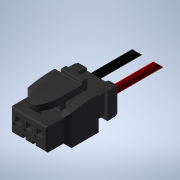
# Autodesk Inventor part: 566654 NEBV-H1G2-KN-0.5-N-LE2
Saved by Autodesk Inventor 2021 (Build 250183000, 183)
## iProperties
Created: 2026-04-16
Part Number: 566654 NEBV-H1G2-KN-0.5-N-LE2
Material: Generic
Catalog Web Link: www.3dfindit.com
Description: NEBV-Connecting cables for valve terminals
Vendor: FESTO
Document SubType Name: Modeling
Designer: psAdmin
Manufacturer: FESTO
Mass: 4 g
Surface Area: 6.95901 cm^2
Volume: 0.50983 cm^3
Density: 1 g/cm^3
Appearance: PSOLRGB-176-176-176
Category: PARTsolutions
Company: FESTO
Title: 566654 NEBV-H1G2-KN-0.5-N-LE2
Author: Cadenas PARTsolutions
Comments: Connecting cables for valve terminals
PSOL_IDENT_0: {$CADENAS_DATA/23d-libs/festo/parts/n/nebv/nebv.prj},197 {VTYP=3D},{NB=566654 NEBV-H1G2-KN-0.5-N-LE2
PSOL_IDENT_1: },{LINA=566654 NEBV-H1G2-KN-0.5-N-LE2},{NN=NEBV},{DATE=23.10.2025 07:10:51},{GEOMDATE=23.10.2025 07:
PSOL_IDENT_2: 10:27},{VERSION=},{LINEID=410},{WBVAR=},{WBNUMERIC=}  {NB=566654 NEBV-H1G2-KN-0.5-N-LE2},{LINA=56665
PSOL_IDENT_3: 4 NEBV-H1G2-KN-0.5-N-LE2},{KT=DUMMY},{TNR=566654},{TYP=NEBV-H1G2-KN-0.5-N-LE2},{INFO=},{KD=0.000},{M
PSOL_IDENT_4: P=-},{L1=0.500},{L2=-},{L3=0.000},{L4=-},{VERS=8},{CNSMASSEXACT=0.0040},{ISASM=0},{PIN=-},{EOLDATE=}
PSOL_IDENT_5: ,{GTIN=4052568057312}
NB: 566654 NEBV-H1G2-KN-0.5-N-LE2
NN: NEBV
NT: Connecting cables for valve terminals
NBSYN: $TNR. $TYP.
LINA: 566654 NEBV-H1G2-KN-0.5-N-LE2
CATALOG: Festo
TNR: 566654
TYP: NEBV-H1G2-KN-0.5-N-LE2
KD: 0
L1: 0.5
L2: -
L3: 0.000
L4: -
CNSMASSEXACT: 0.004
GTIN: 4052568057312
SUPPLIER: FESTO
ARTICLENO: 566654 NEBV-H1G2-KN-0.5-N-LE2
BOMINFO: 566654 NEBV-H1G2-KN-0.5-N-LE2
CREATOR: CADENAS GmbH
Autodesk Inventor part; units mm, degrees
sketch "Sketch_9" plane through (0, 0, 0) normal (1, 0, 0) x (0, 1, 0)
  line L0 (1.4, 13) -> (-2.4, 13)
  line L1 (-2.4, 13) -> (-2.6, 12.8)
  line L2 (-2.6, 12.8) -> (-2.6, 9.85)
  line L3 (-2.6, 9.85) -> (-3.35, 9.1)
  line L4 (-3.35, 9.1) -> (-3.35, 4)
  line L5 (-3.35, 4) -> (-2.07, 4)
  line L6 (-2.07, 4) -> (-2.07, 2)
  line L7 (-2.07, 2) -> (-2.67, 2)
  line L8 (-2.67, 2) -> (-2.6438, 0.5)
  line L9 (-2.6438, 0.5) -> (-2.5098, 0)
  line L10 (-2.5098, 0) -> (2.0698, 0)
  line L11 (2.0698, 0) -> (2.2038, 0.5)
  line L12 (2.2038, 0.5) -> (2.23, 2)
  line L13 (2.23, 2) -> (1.6, 2)
  line L14 (1.6, 2) -> (1.6, 4)
  line L15 (1.6, 4) -> (2.9, 4)
  arc A0 (2.9, 4) -> (2.35, 9.1) centre (-18.6885, 4.2515) ccw
  line L16 (2.35, 9.1) -> (1.6, 9.85)
  line L17 (1.6, 9.85) -> (1.6, 12.8)
  line L18 (1.6, 12.8) -> (1.4, 13)
  constraints: 38 end point, 2 point on circle, 1 centre point
extrude "Extrusion1" add sketch "Sketch_9" along normal mid plane 8.3
sketch "Sketch_23" plane through (0, 0, 0) normal (0, 1, 0) x (-1, 0, 0)
  line L0 (5, 14) -> (-5, 14)
  line L1 (-5, 14) -> (-5, -1)
  line L2 (-5, -1) -> (5, -1)
  line L3 (5, -1) -> (5, 14)
  line L4 (4.13, 9.1) -> (3.38, 9.85)
  line L5 (3.38, 9.85) -> (3.38, 12.8)
  line L6 (3.38, 12.8) -> (3.18, 13)
  line L7 (3.18, 13) -> (-3.18, 13)
  line L8 (-3.18, 13) -> (-3.38, 12.8)
  line L9 (-3.38, 12.8) -> (-3.38, 9.85)
  line L10 (-3.38, 9.85) -> (-4.13, 9.1)
  line L11 (-4.13, 9.1) -> (-4.13, 4)
  line L12 (-4.13, 4) -> (-3.185, 4)
  line L13 (-3.185, 4) -> (-3.185, 2)
  line L14 (-3.185, 2) -> (-3.8, 2)
  line L15 (-3.8, 2) -> (-3.7738, 0.5)
  line L16 (-3.7738, 0.5) -> (-3.6398, 0)
  line L17 (-3.6398, 0) -> (3.6398, 0)
  line L18 (3.6398, 0) -> (3.7738, 0.5)
  line L19 (3.7738, 0.5) -> (3.8, 2)
  line L20 (3.8, 2) -> (3.185, 2)
  line L21 (3.185, 2) -> (3.185, 4)
  line L22 (3.185, 4) -> (4.13, 4)
  line L23 (4.13, 4) -> (4.13, 9.1)
  constraints: 48 end point
extrude "Extrusion2" cut sketch "Sketch_23" along normal mid plane 12
sketch "Sketch_1" plane through (0, 1.6, 0) normal (0, 1, 0) x (1, 0, 0)
  line L0 (-2.8, -4) -> (-2.8, -13)
  line L1 (-2.8, -13) -> (2.8, -13)
  line L2 (2.8, -13) -> (2.8, -4)
  line L3 (2.8, -4) -> (2.04, -4)
  line L4 (2.04, -4) -> (2.04, 0)
  line L5 (2.04, 0) -> (-2.04, 0)
  line L6 (-2.04, 0) -> (-2.04, -4)
  line L7 (-2.04, -4) -> (-2.8, -4)
  constraints: 16 end point
extrude "Extrusion3" cut sketch "Sketch_1" along normal blind 2
sketch "Sketch_2" plane through (0, 0, 0) normal (1, 0, 0) x (0, 1, 0)
  line L0 (3.3881, 12.51) -> (2.87, 12.51)
  line L1 (2.87, 12.51) -> (1.8, 11.6122)
  line L2 (1.8, 11.6122) -> (1.8, 11.3122)
  line L3 (1.8, 11.3122) -> (2.3653, 11.4118)
  arc A0 (2.6, 11.2149) -> (2.3653, 11.4118) centre (2.4, 11.2149) ccw
  line L4 (2.6, 11.2149) -> (2.6, 9.35)
  arc A1 (2.35, 9.1) -> (2.6, 9.35) centre (2.35, 9.35) ccw
  line L5 (2.35, 9.1) -> (1.85, 9.1)
  arc A2 (1.6, 9.35) -> (1.85, 9.1) centre (1.85, 9.35) ccw
  line L6 (1.6, 9.35) -> (0.6, 9.35)
  line L7 (0.6, 9.35) -> (0.6, 7.75)
  line L8 (0.6, 7.75) -> (1.6, 7.75)
  arc A3 (1.95, 8.1) -> (1.6, 7.75) centre (1.95, 7.75) ccw
  line L9 (1.95, 8.1) -> (2.25, 8.1)
  arc A4 (2.6, 7.75) -> (2.25, 8.1) centre (2.25, 7.75) ccw
  line L10 (2.6, 7.75) -> (2.6, 4)
  line L11 (2.6, 4) -> (4.45, 4)
  line L12 (4.45, 4) -> (4.45, 4.8)
  arc A5 (4.45, 4.8) -> (4.25, 5) centre (4.25, 4.8) ccw
  line L13 (4.25, 5) -> (4, 5)
  arc A6 (3.85, 5.15) -> (4, 5) centre (4, 5.15) ccw
  line L14 (3.85, 5.15) -> (3.85, 9.1)
  arc A7 (3.85, 9.1) -> (3.5854, 12.3424) centre (-16.15, 9.1) ccw
  arc A8 (3.5854, 12.3424) -> (3.3881, 12.51) centre (3.3881, 12.31) ccw
  constraints: 30 end point, 18 point on circle, 9 centre point
extrude "Extrusion4" add sketch "Sketch_2" along normal mid plane 4
sketch "Sketch_3" plane through (0, 1.6, 0) normal (0, 1, 0) x (1, 0, 0)
  line L0 (-2.2, -12.8) -> (2.2, -12.8)
  line L1 (2.2, -12.8) -> (2.2, -3.8)
  line L2 (2.2, -3.8) -> (-2.2, -3.8)
  line L3 (-2.2, -3.8) -> (-2.2, -12.8)
  arc A0 (-2, -9.1) -> (-1.1898, -11.8286) centre (3, -9.1) ccw
  arc A1 (-1.1898, -11.8286) -> (1.1898, -11.8286) centre (0, -11.11) ccw
  arc A2 (1.1898, -11.8286) -> (2, -9.1) centre (-3, -9.1) ccw
  line L4 (2, -9.1) -> (2, -4)
  line L5 (2, -4) -> (-2, -4)
  line L6 (-2, -4) -> (-2, -9.1)
  constraints: 14 end point, 6 point on circle, 3 centre point
extrude "Extrusion5" cut sketch "Sketch_3" along normal blind 3
sketch "Sketch_4" plane through (0, 1.6, 0) normal (0, 1, 0) x (1, 0, 0)
  line L0 (-2, -10.5) -> (-2, -13)
  line L1 (-2, -13) -> (-0.765, -13)
  line L2 (-0.765, -13) -> (-0.765, -10.7)
  line L3 (-0.765, -10.7) -> (0.765, -10.7)
  line L4 (0.765, -10.7) -> (0.765, -13)
  line L5 (0.765, -13) -> (2, -13)
  line L6 (2, -13) -> (2, -10.5)
  line L7 (2, -10.5) -> (0.765, -10.5)
  line L8 (0.765, -10.5) -> (0.765, -4)
  line L9 (0.765, -4) -> (2, -4)
  line L10 (2, -4) -> (2, -3)
  line L11 (2, -3) -> (-2, -3)
  line L12 (-2, -3) -> (-2, -4)
  line L13 (-2, -4) -> (-0.765, -4)
  line L14 (-0.765, -4) -> (-0.765, -10.5)
  line L15 (-0.765, -10.5) -> (-2, -10.5)
  constraints: 32 end point
extrude "Extrusion6" cut sketch "Sketch_4" along normal blind 1
sketch "Sketch_5" plane through (0, 0, 4) normal (0, 0, 1) x (1, 0, 0)
  line L0 (-2.3, -3.35) -> (-2.1906, -3.35)
  arc A0 (-1.9953, -3.5068) -> (-2.1906, -3.35) centre (-2.1906, -3.55) ccw
  arc A1 (-1.9953, -3.5068) -> (-1.8621, -3.6537) centre (-1.8, -3.4636) ccw
  arc A2 (-1.8621, -3.6537) -> (1.8621, -3.6537) centre (0, 2.05) ccw
  arc A3 (1.8621, -3.6537) -> (1.9953, -3.5068) centre (1.8, -3.4636) ccw
  arc A4 (2.1906, -3.35) -> (1.9953, -3.5068) centre (2.1906, -3.55) ccw
  line L1 (2.1906, -3.35) -> (2.3, -3.35)
  line L2 (2.3, -3.35) -> (2, 0)
  line L3 (2, 0) -> (-2, 0)
  line L4 (-2, 0) -> (-2.3, -3.35)
  constraints: 10 end point, 10 point on circle, 5 centre point
extrude "Extrusion7" add sketch "Sketch_5" along normal blind 1
sketch "Sketch_6" plane through (0, 0, 9.85) normal (0, 0, 1) x (1, 0, 0)
  line L0 (-1.275, -1.81) -> (-1.275, -3.41)
  line L1 (-1.275, -3.41) -> (1.275, -3.41)
  line L2 (1.275, -3.41) -> (1.275, -1.81)
  line L3 (1.275, -1.81) -> (0.625, -1.81)
  line L4 (0.625, -1.81) -> (0.625, -2.61)
  line L5 (0.625, -2.61) -> (-0.625, -2.61)
  line L6 (-0.625, -2.61) -> (-0.625, -1.81)
  line L7 (-0.625, -1.81) -> (-1.275, -1.81)
  constraints: 16 end point
extrude "Extrusion8" cut sketch "Sketch_6" along normal blind 3.2
sketch "Sketch_19" plane through (0, 0, 13) normal (0, 0, 1) x (1, 0, 0)
  line L0 (-2.4, 0.39) -> (-2.4, -0.41)
  line L1 (-2.4, -0.41) -> (-1.6, -0.41)
  line L2 (-1.6, -0.41) -> (-1.6, 0.39)
  line L3 (-1.6, 0.39) -> (-2.4, 0.39)
  constraints: 8 end point
extrude "Extrusion9" cut sketch "Sketch_19" against normal blind 2.9
sketch "Sketch_20" plane through (0, 0, 13) normal (0, 0, 1) x (1, 0, 0)
  line L0 (-0.4, 0.39) -> (-0.4, -0.41)
  line L1 (-0.4, -0.41) -> (0.4, -0.41)
  line L2 (0.4, -0.41) -> (0.4, 0.39)
  line L3 (0.4, 0.39) -> (-0.4, 0.39)
  constraints: 8 end point
extrude "Extrusion10" cut sketch "Sketch_20" against normal blind 2.9
sketch "Sketch_21" plane through (0, 0, 13) normal (0, 0, 1) x (1, 0, 0)
  line L0 (1.6, 0.39) -> (1.6, -0.41)
  line L1 (1.6, -0.41) -> (2.4, -0.41)
  line L2 (2.4, -0.41) -> (2.4, 0.39)
  line L3 (2.4, 0.39) -> (1.6, 0.39)
  constraints: 8 end point
extrude "Extrusion11" cut sketch "Sketch_21" against normal blind 2.9
sketch "Sketch_7" plane through (0, 0, 13) normal (0, 0, 1) x (1, 0, 0)
  arc A0 (-2.9964, -0.76) -> (-2.0036, -0.76) centre (-2.5, -0.7) ccw
  line L0 (-2.0036, -0.76) -> (-2.9964, -0.76)
  constraints: 2 end point, 2 point on circle, 1 centre point
extrude "Extrusion12" cut sketch "Sketch_7" against normal blind 2.9
sketch "Sketch_8" plane through (0, 0, 13) normal (0, 0, 1) x (1, 0, 0)
  line L0 (0.0036, 0.76) -> (0.9964, 0.76)
  arc A0 (0.9964, 0.76) -> (0.0036, 0.76) centre (0.5, 0.7) ccw
  constraints: 2 end point, 2 point on circle, 1 centre point
extrude "Extrusion13" cut sketch "Sketch_8" against normal blind 2.9
sketch "Sketch_10" plane through (0, 0, 13) normal (0, 0, 1) x (1, 0, 0)
  line L0 (2.0036, 0.76) -> (2.9964, 0.76)
  arc A0 (2.9964, 0.76) -> (2.0036, 0.76) centre (2.5, 0.7) ccw
  constraints: 2 end point, 2 point on circle, 1 centre point
extrude "Extrusion14" cut sketch "Sketch_10" against normal blind 2.9
sketch "Sketch_11" plane through (0, 0, 13) normal (0, 0, 1) x (1, 0, 0)
  line L0 (-1.9964, 0.76) -> (-1.0036, 0.76)
  arc A0 (-1.0036, 0.76) -> (-1.9964, 0.76) centre (-1.5, 0.7) ccw
  constraints: 2 end point, 2 point on circle, 1 centre point
extrude "Extrusion15" cut sketch "Sketch_11" against normal blind 2.9
sketch "Sketch_12" plane through (0, 0, 13) normal (0, 0, 1) x (1, 0, 0)
  arc A0 (-0.9964, -0.76) -> (-0.0036, -0.76) centre (-0.5, -0.7) ccw
  line L0 (-0.0036, -0.76) -> (-0.9964, -0.76)
  constraints: 2 end point, 2 point on circle, 1 centre point
extrude "Extrusion16" cut sketch "Sketch_12" against normal blind 2.9
sketch "Sketch_13" plane through (0, 0, 13) normal (0, 0, 1) x (1, 0, 0)
  arc A0 (1.0036, -0.76) -> (1.9964, -0.76) centre (1.5, -0.7) ccw
  line L0 (1.9964, -0.76) -> (1.0036, -0.76)
  constraints: 2 end point, 2 point on circle, 1 centre point
extrude "Extrusion17" cut sketch "Sketch_13" against normal blind 2.9
sketch "Sketch_14" plane through (0, -0.56, 0) normal (0, 1, 0) x (1, 0, 0)
  line L0 (-2.55, -13) -> (-2.55, -13.5)
  line L1 (-2.55, -13.5) -> (2.55, -13.5)
  line L2 (2.55, -13.5) -> (2.55, -13)
  line L3 (2.55, -13) -> (2.05, -12.5)
  line L4 (2.05, -12.5) -> (1.95, -12.5)
  line L5 (1.95, -12.5) -> (1.45, -13)
  line L6 (1.45, -13) -> (0.55, -13)
  line L7 (0.55, -13) -> (0.05, -12.5)
  line L8 (0.05, -12.5) -> (-0.05, -12.5)
  line L9 (-0.05, -12.5) -> (-0.55, -13)
  line L10 (-0.55, -13) -> (-1.45, -13)
  line L11 (-1.45, -13) -> (-1.95, -12.5)
  line L12 (-1.95, -12.5) -> (-2.05, -12.5)
  line L13 (-2.05, -12.5) -> (-2.55, -13)
  constraints: 28 end point
extrude "Extrusion18" cut sketch "Sketch_14" along normal blind 1.1
sketch "Sketch_15" plane through (0, 0, 0) normal (1, 0, 0) x (0, 1, 0)
  line L0 (0.54, 13) -> (0.39, 12.85)
  line L1 (0.39, 12.85) -> (0.39, 8.1)
  line L2 (0.39, 8.1) -> (-0.41, 8.1)
  line L3 (-0.41, 8.1) -> (-0.41, 12.85)
  line L4 (-0.41, 12.85) -> (-0.56, 13)
  line L5 (-0.56, 13) -> (-0.56, 8)
  line L6 (-0.56, 8) -> (0.54, 8)
  line L7 (0.54, 8) -> (0.54, 13)
  constraints: 16 end point
extrude "Extrusion19" add sketch "Sketch_15" along normal mid plane 6
sketch "Sketch_16" plane through (0, 0, 0) normal (0, 0, 1) x (1, 0, 0)
  circle A0 centre (2, 0) radius 0.65
  constraints: 1 centre point
extrude "Extrusion20" add sketch "Sketch_16" against normal blind 10
sketch "Sketch_17" plane through (0, 0, 0) normal (0, 0, 1) x (1, 0, 0)
  circle A0 centre (-2, 0) radius 0.65
  constraints: 1 centre point
extrude "Extrusion21" add sketch "Sketch_17" against normal blind 10
sketch "Sketch_18" plane through (0, 0, 0) normal (1, 0, 0) x (0, 1, 0)
  line L0 (0.85, -8.5) -> (-0.65, -10)
  line L1 (-0.65, -10) -> (0.85, -10)
  line L2 (0.85, -10) -> (0.85, -8.5)
  constraints: 6 end point
extrude "Extrusion22" cut sketch "Sketch_18" along normal mid plane 6
ref_plane "ANBAU_XY" through (0, 0, 13) normal (0, 0, -1) x (1, 0, 0)
ref_plane "ANBAU_YZ" through (0, 0, 13) normal (1, 0, 0) x (0, -1, 0)
ref_plane "ANBAU_ZX" through (0, 0, 13) normal (0, -1, 0) x (0, 0, -1)
ref_plane "NEBV_XY" through (0, 0.1, 13) normal (0, 0, 1) x (1, 0, 0)
ref_plane "NEBV_YZ" through (0, 0.1, 13) normal (1, 0, 0) x (0, 1, 0)
ref_plane "NEBV_ZX" through (0, 0.1, 13) normal (0, 1, 0) x (0, 0, 1)
body "Solid1"
